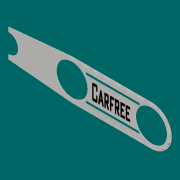
# Autodesk Inventor part: tandem_chain_guard
Saved by Autodesk Inventor 2016 (Build 200138000, 138)
## iProperties
Created: 2016-11-25
Part Number: tandem_chain_guard
Material: Generic
Document SubType Name: Sheet Metal
Designer: katzchristy
Density: 1 g/cm^3
Sheet Metal Rule: Default
Appearance: Default
Author: katzchristy
Autodesk Inventor part; units mm, degrees
ref_plane "YZ Plane" through (0, 0, 0) normal (1, 0, 0) x (0, 1, 0)
ref_plane "XZ Plane" through (0, 0, 0) normal (0, 1, 0) x (-1, 0, 0)
ref_plane "XY Plane" through (0, 0, 0) normal (0, 0, 1) x (1, 0, 0)
sketch "Sketch1" plane through (0, 0, 0) normal (0, 0, 1) x (1, 0, 0)
  circle A0 centre (0, 0) radius 101.6
  circle A1 centre (-508, 0) radius 101.6
  arc A2 (-914.4, -63.5) -> (-914.4, 63.5) centre (-914.4, 0) ccw
  arc A3 (0, -127) -> (0, 127) centre (0, 0) ccw
  line L0 (-508, 127) -> (0, 127)
  line L1 (-508, -127) -> (0, -127)
  line L2 (-914.4, 88.9) -> (-508, 127)
  line L3 (-914.4, -88.9) -> (-508, -127)
  arc A4 (-531.605, -124.787) -> (-508, -127) centre (-508, 0) ccw
  arc A5 (-508, 127) -> (-531.605, 124.787) centre (-508, 0) ccw
  line L4 (-914.4, 88.9) -> (-914.4, 63.5)
  line L5 (-914.4, -63.5) -> (-914.4, -88.9)
  arc A6 (24.7847, 115.2043) -> (-24.7649, 115.2053) centre (0.0093, 84.9651) ccw
  line L6 (21.7734, 111.5288) -> (24.7847, 115.2043)
  line L7 (0, 116.6227) -> (-2.2652, 113.2467)
  line L8 (-2.2652, 113.2467) -> (-6.5296, 113.2467)
  line L9 (-6.5296, 113.2467) -> (-2.6665, 110.2122)
  line L10 (-2.6665, 110.2122) -> (-4.3974, 106.7167)
  line L11 (-4.3974, 106.7167) -> (0, 109.6041)
  line L12 (0, 116.6227) -> (2.2652, 113.2467)
  line L13 (2.2652, 113.2467) -> (6.5296, 113.2467)
  line L14 (6.5296, 113.2467) -> (2.6665, 110.2122)
  line L15 (2.6665, 110.2122) -> (4.3974, 106.7167)
  line L16 (4.3974, 106.7167) -> (0, 109.6041)
  arc A7 (21.7734, 111.5288) -> (-24.7649, 115.2053) centre (-4.6598, 73.316) ccw
  circle A8 centre (27.0709, 110.2598) radius 2.9886
  line L17 (62.6239, 90.7309) -> (59.1689, 88.9203)
  line L18 (61.2821, 95.4565) -> (62.6239, 90.7309)
  line L19 (64.7322, 92.9499) -> (61.2821, 95.4565)
  line L20 (59.1689, 88.9203) -> (64.4237, 88.6716)
  line L21 (68.5491, 94.3498) -> (64.7322, 92.9499)
  line L22 (66.2841, 83.7509) -> (64.4237, 88.6716)
  line L23 (66.9384, 87.5962) -> (66.2841, 83.7509)
  line L24 (68.3973, 90.2871) -> (71.8473, 87.7805)
  line L25 (71.8473, 87.7805) -> (66.9384, 87.5962)
  arc A9 (83.17, 77.4307) -> (47.6808, 107.7595) centre (39.3242, 62.0528) ccw
  arc A10 (87.7666, 78.6341) -> (47.6808, 107.7595) centre (49.9487, 68.7327) ccw
  line L26 (83.17, 77.4307) -> (87.7666, 78.6341)
  circle A11 centre (86.7099, 73.2902) radius 2.9886
  line L27 (68.5491, 94.3498) -> (68.3973, 90.2871)
  line L28 (103.994, 36.5934) -> (100.1347, 37.1594)
  line L29 (105.6862, 41.2052) -> (103.994, 36.5934)
  line L30 (107.004, 37.1494) -> (105.6862, 41.2052)
  line L31 (100.1347, 37.1594) -> (104.2397, 33.8695)
  line L32 (110.9148, 36.0384) -> (107.004, 37.1494)
  line L33 (102.8525, 28.7951) -> (104.2397, 33.8695)
  line L34 (105.642, 31.5214) -> (102.8525, 28.7951)
  line L35 (108.404, 32.8409) -> (109.7217, 28.7851)
  line L36 (109.7217, 28.7851) -> (105.642, 31.5214)
  arc A12 (112.7986, 13.7566) -> (101.914, 59.1532) centre (68.2877, 27.0876) ccw
  arc A13 (117.2247, 12.0284) -> (101.914, 59.1532) centre (80.8095, 26.2468) ccw
  line L37 (112.7986, 13.7566) -> (117.2247, 12.0284)
  circle A14 centre (113.2287, 8.3262) radius 2.9886
  line L38 (110.9148, 36.0384) -> (108.404, 32.8409)
  line L39 (105.642, -31.5214) -> (102.8525, -28.7951)
  line L40 (109.7217, -28.7851) -> (105.642, -31.5214)
  line L41 (108.404, -32.8409) -> (109.7217, -28.7851)
  line L42 (102.8525, -28.7951) -> (104.2397, -33.8695)
  line L43 (110.9148, -36.0384) -> (108.404, -32.8409)
  line L44 (100.1347, -37.1594) -> (104.2397, -33.8695)
  line L45 (103.994, -36.5934) -> (100.1347, -37.1594)
  line L46 (107.004, -37.1494) -> (105.6862, -41.2052)
  line L47 (105.6862, -41.2052) -> (103.994, -36.5934)
  arc A15 (99.3419, -55.172) -> (117.2195, -12.0476) centre (71.1676, -18.2242) ccw
  arc A16 (101.9069, -59.1717) -> (117.2195, -12.0476) centre (80.8037, -26.2645) ccw
  line L48 (99.3419, -55.172) -> (101.9069, -59.1717)
  circle A17 centre (96.4979, -59.8181) radius 2.9886
  line L49 (110.9148, -36.0384) -> (107.004, -37.1494)
  line L50 (66.9384, -87.5962) -> (66.2841, -83.7509)
  line L51 (71.8473, -87.7805) -> (66.9384, -87.5962)
  line L52 (68.3973, -90.2871) -> (71.8473, -87.7805)
  line L53 (66.2841, -83.7509) -> (64.4237, -88.6716)
  line L54 (68.5491, -94.3498) -> (68.3973, -90.2871)
  line L55 (59.1689, -88.9203) -> (64.4237, -88.6716)
  line L56 (62.6239, -90.7309) -> (59.1689, -88.9203)
  line L57 (64.7322, -92.9499) -> (61.2821, -95.4565)
  line L58 (61.2821, -95.4565) -> (62.6239, -90.7309)
  arc A18 (47.94, -103.0268) -> (87.7512, -78.6466) centre (46.8639, -56.5749) ccw
  arc A19 (47.6641, -107.7703) -> (87.7512, -78.6466) centre (49.9337, -68.7436) ccw
  line L59 (47.94, -103.0268) -> (47.6641, -107.7703)
  circle A20 centre (42.9083, -105.1139) radius 2.9886
  line L60 (68.5491, -94.3498) -> (64.7322, -92.9499)
  line L61 (2.6665, -110.2122) -> (4.3974, -106.7167)
  line L62 (6.5296, -113.2467) -> (2.6665, -110.2122)
  line L63 (2.2652, -113.2467) -> (6.5296, -113.2467)
  line L64 (4.3974, -106.7167) -> (0, -109.6041)
  line L65 (0, -116.6227) -> (2.2652, -113.2467)
  line L66 (-4.3974, -106.7167) -> (0, -109.6041)
  line L67 (-2.6665, -110.2122) -> (-4.3974, -106.7167)
  line L68 (-2.2652, -113.2467) -> (-6.5296, -113.2467)
  line L69 (-6.5296, -113.2467) -> (-2.6665, -110.2122)
  arc A21 (-21.7734, -111.5288) -> (24.7649, -115.2053) centre (4.6598, -73.316) ccw
  arc A22 (-24.7847, -115.2043) -> (24.7649, -115.2053) centre (-0.0093, -84.9651) ccw
  line L70 (-21.7734, -111.5288) -> (-24.7847, -115.2043)
  circle A23 centre (-27.0709, -110.2598) radius 2.9886
  line L71 (0, -116.6227) -> (-2.2652, -113.2467)
  line L72 (0, 27.0859) -> (0, -27.0859) construction
  line L73 (-71.12, 27.0859) -> (-71.12, -27.0859) construction
  arc A24 (-46.3353, 115.2043) -> (-95.8849, 115.2053) centre (-71.1107, 84.9651) ccw
  line L74 (-49.3466, 111.5288) -> (-46.3353, 115.2043)
  line L75 (-71.12, 116.6227) -> (-73.3852, 113.2467)
  line L76 (-73.3852, 113.2467) -> (-77.6496, 113.2467)
  line L77 (-77.6496, 113.2467) -> (-73.7865, 110.2122)
  line L78 (-73.7865, 110.2122) -> (-75.5174, 106.7167)
  line L79 (-75.5174, 106.7167) -> (-71.12, 109.6041)
  line L80 (-71.12, 116.6227) -> (-68.8548, 113.2467)
  line L81 (-68.8548, 113.2467) -> (-64.5904, 113.2467)
  line L82 (-64.5904, 113.2467) -> (-68.4535, 110.2122)
  line L83 (-68.4535, 110.2122) -> (-66.7226, 106.7167)
  line L84 (-66.7226, 106.7167) -> (-71.12, 109.6041)
  circle A25 centre (-44.0491, 110.2598) radius 2.9886
  arc A26 (-49.3466, 111.5288) -> (-95.8849, 115.2053) centre (-75.7798, 73.316) ccw
  line L85 (-142.24, 27.0859) -> (-142.24, -27.0859) construction
  arc A27 (-117.4553, 115.2043) -> (-167.0049, 115.2053) centre (-142.2307, 84.9651) ccw
  line L86 (-120.4666, 111.5288) -> (-117.4553, 115.2043)
  line L87 (-142.24, 116.6227) -> (-144.5052, 113.2467)
  line L88 (-144.5052, 113.2467) -> (-148.7696, 113.2467)
  line L89 (-148.7696, 113.2467) -> (-144.9065, 110.2122)
  line L90 (-144.9065, 110.2122) -> (-146.6374, 106.7167)
  line L91 (-146.6374, 106.7167) -> (-142.24, 109.6041)
  line L92 (-142.24, 116.6227) -> (-139.9748, 113.2467)
  line L93 (-139.9748, 113.2467) -> (-135.7104, 113.2467)
  line L94 (-135.7104, 113.2467) -> (-139.5735, 110.2122)
  line L95 (-139.5735, 110.2122) -> (-137.8426, 106.7167)
  line L96 (-137.8426, 106.7167) -> (-142.24, 109.6041)
  circle A28 centre (-115.1691, 110.2598) radius 2.9886
  arc A29 (-120.4666, 111.5288) -> (-167.0049, 115.2053) centre (-146.8998, 73.316) ccw
  line L97 (-213.36, 27.0859) -> (-213.36, -27.0859) construction
  arc A30 (-188.5753, 115.2043) -> (-238.1249, 115.2053) centre (-213.3507, 84.9651) ccw
  line L98 (-191.5866, 111.5288) -> (-188.5753, 115.2043)
  line L99 (-213.36, 116.6227) -> (-215.6252, 113.2467)
  line L100 (-215.6252, 113.2467) -> (-219.8896, 113.2467)
  line L101 (-219.8896, 113.2467) -> (-216.0265, 110.2122)
  line L102 (-216.0265, 110.2122) -> (-217.7574, 106.7167)
  line L103 (-217.7574, 106.7167) -> (-213.36, 109.6041)
  line L104 (-213.36, 116.6227) -> (-211.0948, 113.2467)
  line L105 (-211.0948, 113.2467) -> (-206.8304, 113.2467)
  line L106 (-206.8304, 113.2467) -> (-210.6935, 110.2122)
  line L107 (-210.6935, 110.2122) -> (-208.9626, 106.7167)
  line L108 (-208.9626, 106.7167) -> (-213.36, 109.6041)
  circle A31 centre (-186.2891, 110.2598) radius 2.9886
  arc A32 (-191.5866, 111.5288) -> (-238.1249, 115.2053) centre (-218.0198, 73.316) ccw
  line L109 (-284.48, 27.0859) -> (-284.48, -27.0859) construction
  arc A33 (-259.6953, 115.2043) -> (-309.2449, 115.2053) centre (-284.4707, 84.9651) ccw
  line L110 (-262.7066, 111.5288) -> (-259.6953, 115.2043)
  line L111 (-284.48, 116.6227) -> (-286.7452, 113.2467)
  line L112 (-286.7452, 113.2467) -> (-291.0096, 113.2467)
  line L113 (-291.0096, 113.2467) -> (-287.1465, 110.2122)
  line L114 (-287.1465, 110.2122) -> (-288.8774, 106.7167)
  line L115 (-288.8774, 106.7167) -> (-284.48, 109.6041)
  line L116 (-284.48, 116.6227) -> (-282.2148, 113.2467)
  line L117 (-282.2148, 113.2467) -> (-277.9504, 113.2467)
  line L118 (-277.9504, 113.2467) -> (-281.8135, 110.2122)
  line L119 (-281.8135, 110.2122) -> (-280.0826, 106.7167)
  line L120 (-280.0826, 106.7167) -> (-284.48, 109.6041)
  circle A34 centre (-257.4091, 110.2598) radius 2.9886
  arc A35 (-262.7066, 111.5288) -> (-309.2449, 115.2053) centre (-289.1398, 73.316) ccw
  line L121 (-355.6, 27.0859) -> (-355.6, -27.0859) construction
  arc A36 (-330.8153, 115.2043) -> (-380.3649, 115.2053) centre (-355.5907, 84.9651) ccw
  line L122 (-333.8266, 111.5288) -> (-330.8153, 115.2043)
  line L123 (-355.6, 116.6227) -> (-357.8652, 113.2467)
  line L124 (-357.8652, 113.2467) -> (-362.1296, 113.2467)
  line L125 (-362.1296, 113.2467) -> (-358.2665, 110.2122)
  line L126 (-358.2665, 110.2122) -> (-359.9974, 106.7167)
  line L127 (-359.9974, 106.7167) -> (-355.6, 109.6041)
  line L128 (-355.6, 116.6227) -> (-353.3348, 113.2467)
  line L129 (-353.3348, 113.2467) -> (-349.0704, 113.2467)
  line L130 (-349.0704, 113.2467) -> (-352.9335, 110.2122)
  line L131 (-352.9335, 110.2122) -> (-351.2026, 106.7167)
  line L132 (-351.2026, 106.7167) -> (-355.6, 109.6041)
  circle A37 centre (-328.5291, 110.2598) radius 2.9886
  arc A38 (-333.8266, 111.5288) -> (-380.3649, 115.2053) centre (-360.2598, 73.316) ccw
  line L133 (-426.72, 27.0859) -> (-426.72, -27.0859) construction
  arc A39 (-401.9353, 115.2043) -> (-451.4849, 115.2053) centre (-426.7107, 84.9651) ccw
  line L134 (-404.9466, 111.5288) -> (-401.9353, 115.2043)
  line L135 (-426.72, 116.6227) -> (-428.9852, 113.2467)
  line L136 (-428.9852, 113.2467) -> (-433.2496, 113.2467)
  line L137 (-433.2496, 113.2467) -> (-429.3865, 110.2122)
  line L138 (-429.3865, 110.2122) -> (-431.1174, 106.7167)
  line L139 (-431.1174, 106.7167) -> (-426.72, 109.6041)
  line L140 (-426.72, 116.6227) -> (-424.4548, 113.2467)
  line L141 (-424.4548, 113.2467) -> (-420.1904, 113.2467)
  line L142 (-420.1904, 113.2467) -> (-424.0535, 110.2122)
  line L143 (-424.0535, 110.2122) -> (-422.3226, 106.7167)
  line L144 (-422.3226, 106.7167) -> (-426.72, 109.6041)
  circle A40 centre (-399.6491, 110.2598) radius 2.9886
  arc A41 (-404.9466, 111.5288) -> (-451.4849, 115.2053) centre (-431.3798, 73.316) ccw
  arc A42 (-483.2644, 115.764) -> (-532.8139, 115.765) centre (-508.0398, 85.5248) ccw
  line L145 (-486.2757, 112.0885) -> (-483.2644, 115.764)
  line L146 (-508.049, 117.1824) -> (-510.3142, 113.8064)
  line L147 (-510.3142, 113.8064) -> (-514.5787, 113.8064)
  line L148 (-514.5787, 113.8064) -> (-510.7155, 110.7719)
  line L149 (-510.7155, 110.7719) -> (-512.4464, 107.2764)
  line L150 (-512.4464, 107.2764) -> (-508.049, 110.1638)
  line L151 (-508.049, 117.1824) -> (-505.7839, 113.8064)
  line L152 (-505.7839, 113.8064) -> (-501.5194, 113.8064)
  line L153 (-501.5194, 113.8064) -> (-505.3825, 110.7719)
  line L154 (-505.3825, 110.7719) -> (-503.6517, 107.2764)
  line L155 (-503.6517, 107.2764) -> (-508.049, 110.1638)
  circle A43 centre (-480.9781, 110.8195) radius 2.9886
  arc A44 (-486.2757, 112.0885) -> (-532.8139, 115.765) centre (-512.7088, 73.8757) ccw
  line L156 (-68.4535, -110.2122) -> (-66.7226, -106.7167)
  line L157 (-64.5904, -113.2467) -> (-68.4535, -110.2122)
  line L158 (-68.8548, -113.2467) -> (-64.5904, -113.2467)
  line L159 (-66.7226, -106.7167) -> (-71.12, -109.6041)
  line L160 (-71.12, -116.6227) -> (-68.8548, -113.2467)
  line L161 (-71.12, -116.6227) -> (-73.3852, -113.2467)
  line L162 (-75.5174, -106.7167) -> (-71.12, -109.6041)
  line L163 (-73.7865, -110.2122) -> (-75.5174, -106.7167)
  line L164 (-77.6496, -113.2467) -> (-73.7865, -110.2122)
  line L165 (-73.3852, -113.2467) -> (-77.6496, -113.2467)
  arc A45 (-92.8934, -111.5288) -> (-46.3551, -115.2053) centre (-66.4602, -73.316) ccw
  arc A46 (-95.9047, -115.2043) -> (-46.3551, -115.2053) centre (-71.1293, -84.9651) ccw
  line L166 (-92.8934, -111.5288) -> (-95.9047, -115.2043)
  circle A47 centre (-98.1909, -110.2598) radius 2.9886
  line L167 (-139.5735, -110.2122) -> (-137.8426, -106.7167)
  line L168 (-135.7104, -113.2467) -> (-139.5735, -110.2122)
  line L169 (-139.9748, -113.2467) -> (-135.7104, -113.2467)
  line L170 (-137.8426, -106.7167) -> (-142.24, -109.6041)
  line L171 (-142.24, -116.6227) -> (-139.9748, -113.2467)
  line L172 (-142.24, -116.6227) -> (-144.5052, -113.2467)
  line L173 (-146.6374, -106.7167) -> (-142.24, -109.6041)
  line L174 (-144.9065, -110.2122) -> (-146.6374, -106.7167)
  line L175 (-148.7696, -113.2467) -> (-144.9065, -110.2122)
  line L176 (-144.5052, -113.2467) -> (-148.7696, -113.2467)
  arc A48 (-164.0134, -111.5288) -> (-117.4751, -115.2053) centre (-137.5802, -73.316) ccw
  arc A49 (-167.0247, -115.2043) -> (-117.4751, -115.2053) centre (-142.2493, -84.9651) ccw
  line L177 (-164.0134, -111.5288) -> (-167.0247, -115.2043)
  circle A50 centre (-169.3109, -110.2598) radius 2.9886
  line L178 (-210.6935, -110.2122) -> (-208.9626, -106.7167)
  line L179 (-206.8304, -113.2467) -> (-210.6935, -110.2122)
  line L180 (-211.0948, -113.2467) -> (-206.8304, -113.2467)
  line L181 (-208.9626, -106.7167) -> (-213.36, -109.6041)
  line L182 (-213.36, -116.6227) -> (-211.0948, -113.2467)
  line L183 (-213.36, -116.6227) -> (-215.6252, -113.2467)
  line L184 (-217.7574, -106.7167) -> (-213.36, -109.6041)
  line L185 (-216.0265, -110.2122) -> (-217.7574, -106.7167)
  line L186 (-219.8896, -113.2467) -> (-216.0265, -110.2122)
  line L187 (-215.6252, -113.2467) -> (-219.8896, -113.2467)
  arc A51 (-235.1334, -111.5288) -> (-188.5951, -115.2053) centre (-208.7002, -73.316) ccw
  arc A52 (-238.1447, -115.2043) -> (-188.5951, -115.2053) centre (-213.3693, -84.9651) ccw
  line L188 (-235.1334, -111.5288) -> (-238.1447, -115.2043)
  circle A53 centre (-240.4309, -110.2598) radius 2.9886
  line L189 (-281.8135, -110.2122) -> (-280.0826, -106.7167)
  line L190 (-277.9504, -113.2467) -> (-281.8135, -110.2122)
  line L191 (-282.2148, -113.2467) -> (-277.9504, -113.2467)
  line L192 (-280.0826, -106.7167) -> (-284.48, -109.6041)
  line L193 (-284.48, -116.6227) -> (-282.2148, -113.2467)
  line L194 (-284.48, -116.6227) -> (-286.7452, -113.2467)
  line L195 (-288.8774, -106.7167) -> (-284.48, -109.6041)
  line L196 (-287.1465, -110.2122) -> (-288.8774, -106.7167)
  line L197 (-291.0096, -113.2467) -> (-287.1465, -110.2122)
  line L198 (-286.7452, -113.2467) -> (-291.0096, -113.2467)
  arc A54 (-306.2534, -111.5288) -> (-259.7151, -115.2053) centre (-279.8202, -73.316) ccw
  arc A55 (-309.2647, -115.2043) -> (-259.7151, -115.2053) centre (-284.4893, -84.9651) ccw
  line L199 (-306.2534, -111.5288) -> (-309.2647, -115.2043)
  circle A56 centre (-311.5509, -110.2598) radius 2.9886
  line L200 (-352.9335, -110.2122) -> (-351.2026, -106.7167)
  line L201 (-349.0704, -113.2467) -> (-352.9335, -110.2122)
  line L202 (-353.3348, -113.2467) -> (-349.0704, -113.2467)
  line L203 (-351.2026, -106.7167) -> (-355.6, -109.6041)
  line L204 (-355.6, -116.6227) -> (-353.3348, -113.2467)
  line L205 (-355.6, -116.6227) -> (-357.8652, -113.2467)
  line L206 (-359.9974, -106.7167) -> (-355.6, -109.6041)
  line L207 (-358.2665, -110.2122) -> (-359.9974, -106.7167)
  line L208 (-362.1296, -113.2467) -> (-358.2665, -110.2122)
  line L209 (-357.8652, -113.2467) -> (-362.1296, -113.2467)
  arc A57 (-377.3734, -111.5288) -> (-330.8351, -115.2053) centre (-350.9402, -73.316) ccw
  arc A58 (-380.3847, -115.2043) -> (-330.8351, -115.2053) centre (-355.6093, -84.9651) ccw
  line L210 (-377.3734, -111.5288) -> (-380.3847, -115.2043)
  circle A59 centre (-382.6709, -110.2598) radius 2.9886
  line L211 (-424.0535, -110.2122) -> (-422.3226, -106.7167)
  line L212 (-420.1904, -113.2467) -> (-424.0535, -110.2122)
  line L213 (-424.4548, -113.2467) -> (-420.1904, -113.2467)
  line L214 (-422.3226, -106.7167) -> (-426.72, -109.6041)
  line L215 (-426.72, -116.6227) -> (-424.4548, -113.2467)
  line L216 (-426.72, -116.6227) -> (-428.9852, -113.2467)
  line L217 (-431.1174, -106.7167) -> (-426.72, -109.6041)
  line L218 (-429.3865, -110.2122) -> (-431.1174, -106.7167)
  line L219 (-433.2496, -113.2467) -> (-429.3865, -110.2122)
  line L220 (-428.9852, -113.2467) -> (-433.2496, -113.2467)
  arc A60 (-448.4934, -111.5288) -> (-401.9551, -115.2053) centre (-422.0602, -73.316) ccw
  arc A61 (-451.5047, -115.2043) -> (-401.9551, -115.2053) centre (-426.7293, -84.9651) ccw
  line L221 (-448.4934, -111.5288) -> (-451.5047, -115.2043)
  circle A62 centre (-453.7909, -110.2598) radius 2.9886
  line L222 (-417.6762, 52.3694) -> (16.3381, 52.3694) construction
  line L223 (16.3381, 52.3694) -> (16.3381, -104.3551) construction
  line L224 (16.3381, -104.3551) -> (-417.6762, -104.3551) construction
  line L225 (-417.6762, -104.3551) -> (-417.6762, 52.3694) construction
  line L226 (-422.0602, 88.4304) -> (-81.5085, 88.4304)
  line L227 (-81.5085, 69.7267) -> (-422.0602, 69.7267)
  line L228 (-422.0602, 69.7267) -> (-422.0602, 88.4304)
  arc A63 (-66.697, 84.3192) -> (-81.5085, 69.7267) centre (-41.6839, 44.1174) ccw
  line L229 (-81.5085, 88.4304) -> (-66.697, 84.3192)
  line L230 (-380.5348, 0.439) -> (-74.1027, 0.439) construction
  line L231 (-422.0602, -87.5525) -> (-81.5085, -87.5525)
  line L232 (-81.5085, -68.8488) -> (-422.0602, -68.8488)
  line L233 (-422.0602, -68.8488) -> (-422.0602, -87.5525)
  arc A64 (-81.5085, -68.8488) -> (-66.697, -83.4413) centre (-41.6839, -43.2395) ccw
  line L234 (-81.5085, -87.5525) -> (-66.697, -83.4413)
  point P0 (-71.1107, -84.0872)
  point P1 (-75.7798, -72.438)
  point P2 (-142.2307, -84.0872)
  point P3 (-146.8998, -72.438)
  point P4 (-213.3507, -84.0872)
  point P5 (-218.0198, -72.438)
  point P6 (-284.4707, -84.0872)
  point P7 (-289.1398, -72.438)
  point P8 (-355.5907, -84.0872)
  point P9 (-360.2598, -72.438)
  point P10 (-426.7107, -84.0872)
  dimension "d0" = 203.2
  dimension "d1" = 203.2
  dimension "d3" = 127
  dimension "d4" = 406.4
  dimension "d5" = 25.4
  dimension "d11" = 180
  dimension "d15" = 71.12
  dimension "d28" = 71.12
  measures "d0" diameter of A0
  measures "d1" diameter of A1
  measures "d3" diameter of A2
  measures "d4" distance of A1.centre A2.centre
  measures "d5" radial gap between concentric circles of A0 A3
  measures "d15" distance of L72.start L73.start
  measures "d28" distance of A21.end A45.end
extrude "Plate2" add sketch "Sketch1" along normal blind 3.048 contours A2 L4 L2 L0 A3 L1 L3 L5
sketch "Sketch2" plane through (0, 0, 3.048) normal (0, 0, 1) x (1, 0, 0)
  line L0 (-385.4934, 52.2081) -> (-118.9358, 52.2081) construction
  line L1 (-118.9358, 52.2081) -> (-118.9358, -44.8867) construction
  line L2 (-118.9358, -44.8867) -> (-385.4934, -44.8867) construction
  line L3 (-385.4934, -44.8867) -> (-385.4934, 52.2081) construction
  point P0 (0, 0)
  constraints: 2 other
equation "\"d1\" = d0"
equation "\"BendRadius\" = Thickness"
equation "\"BendReliefWidth\" = Thickness"
equation "\"BendReliefDepth\" = 0.5 * Thickness"
equation "\"CornerReliefSize\" = 4 * Thickness"
equation "\"MinimumRemnant\" = 2 * Thickness"
equation "\"TransitionRadius\" = BendRadius"
equation "\"JacobiRadiusSize\" = BendRadius"
equation "\"GapSize\" = Thickness"
equation "\"d8\" = BendRadius"
equation "\"d33\" = BendRadius"
equation "\"Thickness\" = 3.048"
body "Solid2"
